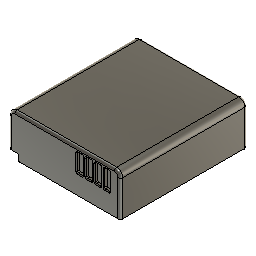
Panasonic DMW-BLG10E battery v1 (Autodesk Fusion 360 design; units mm, degrees)
Autodesk Fusion 360 part; units mm, degrees
note: some values were not read from the file. Chosen so that the rebuilt part matches the saved one: which face or edge a step refers to.
sketch "Sketch1" plane through (0, 0, 0) normal (0, 0, 1) x (1, 0, 0)
  line L0 (0, 0) -> (36.8, 0)
  line L1 (36.8, 0) -> (36.8, 41.84)
  line L2 (36.8, 41.84) -> (0, 41.84)
  line L3 (0, 41.84) -> (0, 0)
  dimension "d1" = 41.84
  dimension "d2" = 36.8
  constraint horizontal L0
  constraint vertical L1
  constraint horizontal L2
  constraint vertical L3
  constraint coincident L0.start L3.end
  measures "d1" distance of L0.start L2.end
  measures "d2" distance of L1.end L2.end
extrude "Extrude1" add sketch "Sketch1" along normal blind 14.15
sketch "Sketch2" plane through (0, 0, 0) normal (0, -1, 0) x (1, 0, 0)
  line L0 (0.8, 0.4) -> (36, 0.4)
  line L1 (36, 0.4) -> (36, 12.15)
  arc A0 (36, 12.15) -> (34.8, 13.35) centre (34.8, 12.15) ccw
  line L2 (34.8, 13.35) -> (2, 13.35)
  arc A1 (2, 13.35) -> (0.8, 12.15) centre (2, 12.15) ccw
  line L3 (0.8, 12.15) -> (0.8, 0.4)
  line L4 (0, 0) -> (3.35, 0)
  line L5 (3.35, 0) -> (3.35, 2.5)
  line L6 (3.35, 2.5) -> (0, 2.5)
  line L7 (0, 2.5) -> (0, 0)
  dimension "d11" = 3.35
  dimension "d12" = 2.5
  constraint horizontal L4
  constraint vertical L5
  constraint horizontal L6
  constraint vertical L7
  constraint coincident L4.start L7.end
  measures "d11" distance of L5.end L6.end
  measures "d12" distance of L4.start L6.end
extrude "Extrude2" cut sketch "Sketch2" against normal blind 3.1 contours L0 L3 L5 L6 | L0 L3 L4 L5 L6 L7
fillet "Fillet1" radius 2 2 edges at (0, 20.92, 14.15) (36.8, 20.92, 14.15)
fillet "Fillet2" radius 0.8 10 edges at (0, 0, 7.325) (0.5858, 0, 13.5642) (18.4, 0, 14.15) (36.2142, 0, 13.5642) (36.8, 0, 6.075) (36.8, 41.84, 6.075) (36.2142, 41.84, 13.5642) (18.4, 41.84, 14.15) (0.5858, 41.84, 13.5642) (0, 41.84, 6.075)
fillet "Fillet3" radius 0.4 7 edges at (0, 22.07, 0) (0.2343, 41.6057, 0) (18.4, 41.84, 0) (36.5657, 41.6057, 0) (36.8, 20.92, 0) (36.5657, 0.2343, 0) (19.675, 0, 0)
sketch "Sketch3" plane through (0, 0, 0) normal (0, -1, 0) x (1, 0, 0)
  line L0 (3.35, 0.4) -> (36, 0.4)
  line L1 (36, 0.4) -> (36, 12.15)
  arc A0 (36, 12.15) -> (34.8, 13.35) centre (34.8, 12.15) ccw
  line L2 (34.8, 13.35) -> (2, 13.35)
  arc A1 (2, 13.35) -> (0.8, 12.15) centre (2, 12.15) ccw
  line L3 (0.8, 12.15) -> (0.8, 2.5)
  line L4 (0.8, 2.5) -> (3.35, 2.5)
  line L5 (3.35, 2.5) -> (3.35, 0.4)
  line L6 (33.4, 12.6491) -> (31.4, 12.6491)
  line L7 (31.4, 12.6491) -> (31.4, 6.6491)
  line L8 (31.4, 6.6491) -> (33.4, 6.6491)
  line L9 (33.4, 6.6491) -> (33.4, 12.6491)
  line L10 (36.8, 0.4) -> (36.8, 12.15)
  line L11 (30.4, 6.7099) -> (28.4, 6.7099)
  line L12 (28.4, 6.7099) -> (28.4, 12.6491)
  line L13 (28.4, 12.6491) -> (30.4, 12.6491)
  line L14 (30.4, 12.6491) -> (30.4, 6.7099)
  line L15 (27.4, 12.6491) -> (25.4, 12.6491)
  line L16 (25.4, 12.6491) -> (25.4, 6.7099)
  line L17 (25.4, 6.7099) -> (27.4, 6.7099)
  line L18 (27.4, 6.7099) -> (27.4, 12.6491)
  line L19 (24.4, 6.7099) -> (22.4, 6.7099)
  line L20 (22.4, 6.7099) -> (22.4, 12.6491)
  line L21 (22.4, 12.6491) -> (24.4, 12.6491)
  line L22 (24.4, 12.6491) -> (24.4, 6.7099)
  dimension "d15" = 2
  dimension "d16" = 3.4
  dimension "d17" = 6
  dimension "d18" = 11
  dimension "d19" = 3
  dimension "d20" = 6
  constraint horizontal L6
  constraint vertical L7
  constraint horizontal L8
  constraint vertical L9
  constraint horizontal L11
  constraint vertical L12
  constraint horizontal L13
  constraint vertical L14
  constraint horizontal L15
  constraint vertical L16
  constraint horizontal L17
  constraint vertical L18
  constraint horizontal L19
  constraint vertical L20
  constraint horizontal L21
  constraint vertical L22
  constraint collinear L6 L13
  constraint collinear L13 L15
  constraint collinear L15 L21
  constraint equal L11 L17
  constraint equal L17 L19
  constraint equal L8 L19
  measures "d15" distance of L6.start L6.end
  measures "d16" distance of L9 L10
  measures "d17" distance of L6.start L8.end
  measures "d18" distance of L9 L20
  measures "d19" distance of L9 L14
  measures "d20" distance of L9 L18
extrude "Extrude3" cut sketch "Sketch3" against normal blind 1 contours L6 L7 L8 L9 | L11 L12 L13 L14 | L15 L16 L17 L18 | L19 L20 L21 L22
fillet "Fillet4" radius 0.3 32 edges at (24.4, 0.5, 6.7099) (27.4, 0.5, 6.7099) (30.4, 0.5, 6.7099) (33.4, 0.5, 6.6491) (33.4, 0.5, 12.6491) (30.4, 0.5, 12.6491) (27.4, 0.5, 12.6491) (24.4, 0.5, 12.6491) (22.4, 0.5, 12.6491) (25.4, 0.5, 12.6491) (28.4, 0.5, 12.6491) (31.4, 0.5, 12.6491) (22.4, 0.5, 6.7099) (25.4, 0.5, 6.7099) (28.4, 0.5, 6.7099) (31.4, 0.5, 6.6491) (31.4, 0, 9.6491) (30.4, 0, 9.6795) (28.4, 0, 9.6795) (29.4, 0, 6.7099) (29.4, 0, 12.6491) (32.4, 0, 12.6491) (33.4, 0, 9.6491) (32.4, 0, 6.6491) (26.4, 0, 6.7099) (27.4, 0, 9.6795) (26.4, 0, 12.6491) (25.4, 0, 9.6795) (24.4, 0, 9.6795) (23.4, 0, 12.6491) (22.4, 0, 9.6795) (23.4, 0, 6.7099)
